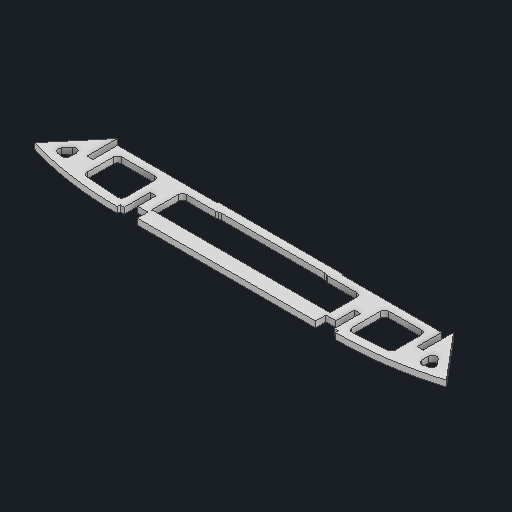
# Autodesk Inventor part: tail_2
Saved by Autodesk Inventor 2024 (Build 280153000, 153)
## iProperties
Created: 2022-03-21
Part Number: tail_2
Material: Generic
Document SubType Name: Modeling
Designer: kardo
Density: 1 g/cm^3
Appearance: Default
Mass: 7.66502 g
Surface Area: 79.4064 cm^2
Volume: 7.66502 cm^3
Author: kardo
Autodesk Inventor part; units mm, degrees
ref_plane "YZ Plane" through (0, 0, 0) normal (1, 0, 0) x (0, 1, 0)
ref_plane "XZ Plane" through (0, 0, 0) normal (0, 1, 0) x (-1, 0, 0)
ref_plane "XY Plane" through (0, 0, 0) normal (0, 0, 1) x (1, 0, 0)
derived "parameters_frame.ipt"
derived "stencil_frame.ipt"
sketch "sk_joint_locations" plane through (81.12, 0, 0) normal (1, 0, 0) x (0, 1, 0)
  line L0 (0, 0) -> (122.4, 9.6331) construction
  line L1 (36.465, 28.832) -> (112.2, 28.832) construction
  arc A0 (36.465, 28.832) -> (11.22, 28.376) centre (36.465, -670.197) ccw construction
  line L2 (-241.5001, 19.2432) -> (11.22, 28.376) construction
  line L3 (-345, 16.32) -> (-262.2001, 18.586) construction
  arc A1 (-262.2001, 18.586) -> (-241.5001, 19.2432) centre (-326.8578, 2381.2399) ccw construction
  line L4 (-122.4795, 3121.122) -> (270.8781, -1876.9598) construction
  line L5 (-230.0001, 3089.1136) -> (-230.0001, -1866.0023) construction
  line L6 (-114.9999, 3089.1136) -> (-114.9999, -1866.0023) construction
  line L7 (-345, 3089.1136) -> (-345, -1866.0023) construction
  line L8 (0, 3089.1136) -> (0, -1866.0023) construction
  line L9 (529.622, 47.2379) -> (-602.608, 2.7525) construction
  line L10 (-673.1615, -36.5999) -> (647.9226, 67.3717) construction
  line L11 (189.4528, 29.5173) -> (189.1111, 38.2146) construction
  line L12 (201.105, 36.5853) -> (201.7901, 27.8813) construction
  line L13 (0, 14.144) -> (121.9006, 15.9783) construction
  line L14 (-230.0001, 45.8224) -> (-230.0001, 19.6588) construction
  line L15 (-345, 37.3935) -> (-345, 16.32) construction
  line L16 (-114.9999, 50.9907) -> (-114.9999, 23.8147) construction
  line L17 (0, 52.89) -> (0, 27.9705) construction
  line L18 (119.1768, 50.5875) -> (119.7216, 43.6656) construction
  line L19 (120.2663, 36.7438) -> (119.7216, 43.6656) construction
  line L20 (120.2663, 36.7438) -> (120.8111, 29.822) construction
  line L21 (120.8111, 29.822) -> (121.3559, 22.9001) construction
  line L22 (121.3559, 22.9001) -> (121.9006, 15.9783) construction
  line L23 (0, 14.144) -> (0, 0) construction
  spline S0 degree 4 poles (-345, 37.3935) (-258.8686, 45.1235) (-172.5923, 49.7074) (-86.3167, 52.89) (0, 52.89) knots 0 0 0 0 0 1 1 1 1 1
  spline S1 degree 3 poles (0, 52.89) (92.8353, 52.89) (195.0311, 49.5089) (255, 36.448) knots 0 0 0 0 1 1 1 1
  spline S2 degree 2 poles (122.4, 9.6331) (190.08, 14.9596) (255, 36.448) knots 0 0 0 1 1 1
  line L24 (112.2, 37.536) -> (112.2, 28.832) construction
  line L25 (112.2, 35.848) -> (112.2, 30.52) construction
  point P0 (-122.4795, 3121.122)
  point P1 (270.8781, -1876.9598)
  point P2 (189.282, 33.8659)
  point P3 (201.4475, 32.2333)
  point P4 (134.9575, 11.3411)
  point P5 (-345, 26.8568)
  point P6 (-230.0001, 32.7406)
  point P7 (-114.9999, 37.4027)
  point P8 (0, 40.4303)
  point P9 (112.2, 33.184)
sketch "sk_cowl_joint_locations" plane through (54.6, 0, 0) normal (1, 0, 0) x (0, 1, 0)
  line L0 (-345, 16.32) -> (-262.2001, 18.586) construction
  arc A0 (-262.2001, 18.586) -> (-241.5001, 19.2432) centre (-326.8578, 2381.2399) ccw construction
  line L1 (-241.5001, 19.2432) -> (11.22, 28.376) construction
  arc A1 (36.465, 28.832) -> (11.22, 28.376) centre (36.465, -670.197) ccw construction
  line L2 (36.465, 28.832) -> (112.2, 28.832) construction
  line L3 (94.8, 29.632) -> (36.465, 29.632) construction
  arc A2 (36.465, 29.632) -> (11.1911, 29.1755) centre (36.465, -670.197) ccw construction
  line L4 (11.1911, 29.1755) -> (-241.529, 20.0427) construction
  arc A3 (-262.222, 19.3857) -> (-241.529, 20.0427) centre (-326.8578, 2381.2399) ccw construction
  line L5 (-262.222, 19.3857) -> (-345, 17.1203) construction
  line L6 (-230.0001, 3089.1136) -> (-230.0001, -1866.0023) construction
  line L7 (-114.9999, 3089.1136) -> (-114.9999, -1866.0023) construction
  line L8 (-345, 3089.1136) -> (-345, -1866.0023) construction
  line L9 (0, 3089.1136) -> (0, -1866.0023) construction
  line L10 (-230.0001, 44.8681) -> (-230.0001, 20.4593) construction
  line L11 (-114.9999, 49.7658) -> (-114.9999, 24.6152) construction
  line L12 (-345, 17.1203) -> (-345, 17.1203)
  line L13 (-345, 17.1203) -> (-345, 36.7228) construction
  line L14 (-850.7464, 3011.9134) -> (325.2296, -1886.3794) construction
  line L15 (-344.7454, 36.7228) -> (-345, 39.712) construction
  line L16 (0, 51.4) -> (0, 28.7711) construction
  spline S0 degree 2 poles (-345, 39.712) (-172.656, 54.3934) (0, 54.4) knots 0 0 0 1 1 1
  spline S1 degree 3 poles (0, 54.4) (37.026, 54.4) (80.784, 47.9917) (112.2, 37.536) knots 1 1 1 1 2 2 2 2
  spline S2 degree 3 poles (111.2526, 34.6895) (106.0906, 36.4075) (96.4401, 39.2282) (84.5011, 42.0313) (75.2591, 43.9395) (68.9709, 45.1125) (60.9945, 46.449) (54.5373, 47.4124) (46.413, 48.4791) (39.8882, 49.2203) (31.7426, 50.0013) (25.2514, 50.5076) (17.2112, 50.9875) (9.2661, 51.3118) (3.0567, 51.4) (0, 51.4) knots 1 1 1 1 1.166667 1.291667 1.333333 1.416667 1.458333 1.541667 1.583333 1.666667 1.708333 1.791667 1.833333 1.916667 2 2 2 2
  spline S3 degree 3 poles (0, 51.4) (-19.1698, 51.3993) (-52.712, 51.1604) (-91.0357, 50.4121) (-119.7742, 49.6473) (-138.931, 49.0355) (-162.8744, 48.1436) (-182.0269, 47.3282) (-205.9648, 46.1816) (-225.113, 45.1626) (-249.0455, 43.7615) (-268.1894, 42.5387) (-292.1166, 40.883) (-316.041, 39.1) (-335.1777, 37.5379) (-344.7454, 36.7228) knots 0 0 0 0 0.166667 0.291667 0.333333 0.416667 0.458333 0.541666 0.583333 0.666666 0.708333 0.791666 0.833333 0.916666 1 1 1 1
  line L17 (-144.5331, 44.6212) -> (-139.5174, 23.7292) construction
  line L18 (-134.9371, 30.3529) -> (-140.7713, 28.9522) construction
  line L19 (-137.4449, 40.7989) -> (-143.2792, 39.3982) construction
  line L20 (-144.5331, 44.6212) -> (-138.6989, 46.0219) construction
  line L21 (-139.5174, 23.7292) -> (-133.6831, 25.1299) construction
  line L22 (-138.6989, 46.0219) -> (-138.9044, 52.0184) construction
  point P0 (0, 0)
  point P1 (-345, 26.9216)
  point P2 (-230.0001, 32.6637)
  point P3 (-114.9999, 37.1905)
  point P4 (0, 40.0855)
  point P5 (-850.7464, 3011.9134)
  point P6 (325.2296, -1886.3794)
  point P7 (-85.2629, 50.788)
  point P8 (0, 40.0855)
sketch "sk_tail_2_base" plane through (0, -230.0001, 0) normal (0, 1, 0) x (-1, 0, 0)
  spline S0 degree 2 poles (-54.6, 47.873) (-109.4, 47.873) (-156, 14.131) knots 0 0 0 1 1 1 construction
  line L0 (0, 47.873) -> (-54.6, 47.873) construction
  line L1 (890.6767, -1145.4489) -> (-1641.6614, 1872.4742) construction
  line L2 (0, -1866.0023) -> (0, 3089.1136) construction
  line L3 (0, 19.8827) -> (-31.32, 19.8827)
  line L4 (-31.32, 19.8827) -> (-31.32, 20.4588)
  line L5 (-31.32, 20.4588) -> (-81.12, 20.4588)
  line L6 (-81.12, 20.4588) -> (-81.12, 32.7406)
  line L7 (-81.12, 32.7406) -> (-84.12, 32.7406)
  line L8 (-84.12, 32.7406) -> (-84.12, 17.5132)
  line L9 (-84.12, 17.5132) -> (-102.9792, 39.9887)
  line L10 (0, 47.073) -> (-54.6, 47.073)
  line L11 (0, 47.073) -> (0, 19.8827)
  spline S1 degree 5 poles (-54.6, 47.073) (-65.2793, 47.0728) (-75.958, 46.2693) (-86.5576, 44.5987) (-107.6468, 39.4344) (-127.6111, 30.8885) (-137.3447, 25.7475) (-146.6519, 19.912) (-155.5308, 13.483) knots 0 0 0 0 0 0 0.493469 0.493469 0.493469 1 1 1 1 1 1
  point P0 (0, 0)
  point P1 (-34.32, 19.6588)
  point P2 (-34.32, 19.0827)
  dimension "d3" = 0.8
  dimension "d4" = 0.8
  dimension "d5" = 0.8
  dimension "d6" = 3
  dimension "d7" = 3
  dimension "d8" = 0.8
  constraints: 18 end point, 5 parallel, 4 perpendicular, 2 point on line, 1 coincident, 4 other
  measures "d4" distance from line of L3 point (-34.32, 19.083)
  measures "d5" distance from line of L5 point (-34.32, 19.659)
  measures "d6" distance from line of point (-34.32, 19.659) L4
  measures "d7" distance of L6.end L7.end
  measures "d8" distance between parallel lines of L1 L9
extrude "thicken" add sketch "sk_tail_2_base" along normal blind 3
sketch "sk_cut_joint" plane through (0, -230.0001, 0) normal (0, 1, 0) x (-1, 0, 0)
  line L0 (0, 47.873) -> (-54.6, 47.873) projected
  line L1 (-54.6, -1866.0023) -> (-54.6, 3089.1136) construction
  line L2 (-49.6, 47.873) -> (-49.6, 32.6637)
  line L3 (-49.6, 32.6637) -> (-52.6, 32.6637)
  line L4 (-52.6, 32.6637) -> (-52.6, 47.873)
  point P0 (0, 0)
  point P1 (-54.6, 32.6637)
  dimension "d11" = 5
  dimension "d12" = 3
  constraints: 6 end point, 3 parallel, 3 point on line
  measures "d11" distance between parallel lines of L1 L2
  measures "d12" distance between parallel lines of L2 L4
extrude "cut_joint" cut sketch "sk_cut_joint" along normal through all both and the other way through all
sketch "sk_cut_liner" plane through (0, -230.0001, 0) normal (0, 1, 0) x (-1, 0, 0)
  line L0 (0, 47.873) -> (-54.6, 47.873) projected
  line L1 (-54.6, -1866.0023) -> (-54.6, 3089.1136) projected
  line L2 (-44.6, 47.873) -> (-44.6, 41.873)
  line L3 (-44.6, 41.873) -> (-49.6, 41.873)
  line L4 (-49.6, 41.873) -> (-49.6, 45.573)
  line L5 (-49.6, 45.573) -> (-54.6, 45.573)
  point P0 (0, 0)
  dimension "d14" = 2.3
  dimension "d15" = 5
  dimension "d17" = 5
  dimension "d40" = 6
  constraints: 8 end point, 4 parallel, 2 point on line
  measures "d14" distance between parallel lines of L0 L5
  measures "d15" distance between parallel lines of L1 L4
  measures "d17" distance between parallel lines of L2 L4
  measures "d40" distance of L2.start L2.end
extrude "cut_liner" cut sketch "sk_cut_liner" along normal through all both and the other way through all
sketch "sk_cut_weight" plane through (0, -230.0001, 0) normal (0, 1, 0) x (-1, 0, 0)
  line L0 (-44.6, 47.873) -> (-44.6, 41.873) construction
  line L1 (-44.6, 41.873) -> (-49.6, 41.873) construction
  line L2 (-49.6, 41.873) -> (-49.6, 45.573) projected
  line L3 (-31.32, 20.4588) -> (-81.12, 20.4588) construction
  line L4 (-31.32, 19.8827) -> (-31.32, 20.4588) construction
  line L5 (0, 19.8827) -> (-31.32, 19.8827) construction
  line L6 (-81.12, 20.4588) -> (-81.12, 32.7406) construction
  line L7 (-84.12, 32.7406) -> (-84.12, 17.5132) construction
  spline S0 degree 3 poles (-54.6, 47.073) (-57.6308, 47.073) (-63.654, 46.9175) (-71.0875, 46.3344) (-78.4496, 45.4599) (-84.2822, 44.5272) (-91.502, 43.0699) (-97.221, 41.6708) (-104.2991, 39.6306) (-109.9051, 37.7651) (-116.8422, 35.1417) (-122.3357, 32.8095) (-130.4917, 28.9611) (-141.2169, 23.207) (-150.3731, 17.2176) (-155.5308, 13.483) knots 0 0 0 0 0.083333 0.166667 0.208333 0.291667 0.333333 0.416667 0.458333 0.541667 0.583333 0.666667 0.708333 0.833333 1 1 1 1 construction
  line L8 (-84.12, 17.5132) -> (-102.9792, 39.9887) construction
  line L9 (0, -1866.0023) -> (0, 3089.1136) projected
  line L10 (-88.12, 28.5031) -> (-88.12, 39.7473)
  line L11 (-88.12, 39.7473) -> (-96.2058, 38.1394)
  line L12 (-96.2058, 38.1394) -> (-88.12, 28.5031)
  line L13 (-88.12, 39.7473) -> (-88.12, 43.7473) construction
  line L14 (-96.2058, 38.1394) -> (-98.777, 41.2036) construction
  line L15 (0, 39.873) -> (-44.6, 39.873)
  line L16 (-44.6, 39.873) -> (-44.6, 24.4588)
  line L17 (-44.6, 24.4588) -> (-27.32, 24.4588)
  line L18 (-27.32, 24.4588) -> (-27.32, 23.8827)
  line L19 (-27.32, 23.8827) -> (0, 23.8827)
  line L20 (-56.6, 43.073) -> (-77.12, 41.5672)
  line L21 (-77.12, 41.5672) -> (-77.12, 24.4588)
  line L22 (-77.12, 24.4588) -> (-56.6, 24.4588)
  line L23 (-56.6, 24.4588) -> (-56.6, 43.073)
  line L24 (-49.6, 41.873) -> (-49.6, 20.4588) construction
  line L25 (-49.6, 41.873) -> (-52.6, 41.873) construction
  line L26 (-52.6, 41.873) -> (-52.6, 20.4588) construction
  line L27 (-77.12, 41.5672) -> (-77.4127, 45.5565) construction
  point P0 (0, 0)
  dimension "d22" = 3
  dimension "d23" = 4
  dimension "d24" = 4
  dimension "d25" = 4
  dimension "d26" = 4
  dimension "d28" = 4
  dimension "d29" = 4
  dimension "d30" = 4
  dimension "d31" = 4
  dimension "d32" = 4
  dimension "d33" = 4
  dimension "d34" = 4
  dimension "d35" = 2
  dimension "d39" = 4
  constraints: 36 end point, 11 parallel, 4 collinear, 4 point on line, 2 perpendicular, 3 other
  measures "d22" distance between parallel lines of L24 L26
  measures "d23" distance between parallel lines of L23 L26
  measures "d24" distance between parallel lines of L3 L22
  measures "d25" distance between parallel lines of L6 L21
  measures "d26" distance of L20.end L27.end
  measures "d28" distance between parallel lines of L7 L10
  measures "d29" distance between parallel lines of L8 L12
  measures "d30" distance of L10.end L13.end
  measures "d31" distance of L11.end L14.end
  measures "d32" distance between parallel lines of L5 L19
  measures "d33" distance between parallel lines of L4 L18
  measures "d34" distance between parallel lines of L3 L17
  measures "d35" distance between parallel lines of L1 L15
  measures "d39" vertical distance of L20.start point (-54.6, 47.073)
extrude "cut_weight" cut sketch "sk_cut_weight" along normal through all both and the other way through all
fillet "rounding" radius 2 10 edges at (27.32, -228.5001, 24.4588) (27.32, -228.5001, 23.8827) (44.6, -228.5001, 24.4588) (77.12, -228.5001, 41.5672) (96.2058, -228.5001, 38.1394) (77.12, -228.5001, 24.4588) (88.12, -228.5001, 28.5031) (56.6, -228.5001, 24.4588) (56.6, -228.5001, 43.073) (88.12, -228.5001, 39.7473)
mirror "mirror" about plane through (0, 0, 0) normal (1, 0, 0)
equation "\"d3\" = shell_thickness"
equation "\"d4\" = shell_thickness"
equation "\"d5\" = shell_thickness"
equation "\"d6\" = bulkhead_thickness"
equation "\"d7\" = stringer_thickness"
equation "\"d8\" = shell_thickness"
equation "\"d9\" = bulkhead_thickness"
equation "\"d11\" = cowl_liner_width"
equation "\"d12\" = bulkhead_thickness"
equation "\"d14\" = shell_thickness + cowl_liner_thickness"
equation "\"d15\" = cowl_liner_width"
equation "\"d17\" = cowl_sealing_width"
equation "\"d40\" = cowl_sealing_thickness + cowl_shell_thickness + cowl_liner_thickness"
equation "\"d22\" = bulkhead_thickness"
equation "\"d23\" = bulkhead_inset"
equation "\"d24\" = bulkhead_inset"
equation "\"d25\" = bulkhead_inset"
equation "\"d26\" = bulkhead_inset"
equation "\"d28\" = bulkhead_inset"
equation "\"d29\" = bulkhead_inset"
equation "\"d30\" = bulkhead_inset"
equation "\"d31\" = bulkhead_inset"
equation "\"d32\" = bulkhead_inset"
equation "\"d33\" = bulkhead_inset"
equation "\"d34\" = bulkhead_inset"
equation "\"d39\" = bulkhead_inset"
equation "\"d38\" = 0.5 * bulkhead_inset"
equation "\"shell_thickness\" = 0.8"
equation "\"stringer_thickness\" = 3"
equation "\"bulkhead_thickness\" = 3"
equation "\"cowl_liner_width\" = 5"
equation "\"cowl_liner_thickness\" = 1.5"
equation "\"cowl_sealing_width\" = 5"
equation "\"cowl_sealing_thickness\" = 3"
equation "\"cowl_shell_thickness\" = 1.5"
equation "\"bulkhead_inset\" = 4"
body "Solid1"
